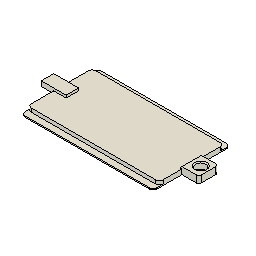
receiver_assembly (Autodesk Fusion 360 archive; units mm, degrees)
design "receiver_battery_door"
Autodesk Fusion 360 part; units mm, degrees
sketch "Sketch1" plane through (0, 0, 0) normal (0, 1, 0) x (1, 0, 0)
  line L0 (26.45, 12.95) -> (-26.45, 12.95)
  line L1 (-26.45, 12.95) -> (-26.45, -12.95)
  line L2 (-26.45, -12.95) -> (26.45, -12.95)
  line L3 (26.45, -12.95) -> (26.45, 12.95)
  line L4 (26.45, 12.95) -> (-26.45, -12.95) construction
  line L5 (-26.45, 12.95) -> (26.45, -12.95) construction
  line L6 (26.45, -15.45) -> (-26.45, -15.45)
  line L7 (-26.45, -15.45) -> (-26.45, 15.45)
  line L8 (-26.45, 15.45) -> (26.45, 15.45)
  line L9 (26.45, 15.45) -> (26.45, -15.45)
  line L10 (26.45, -15.45) -> (-26.45, 15.45) construction
  line L11 (-26.45, -15.45) -> (26.45, 15.45) construction
  dimension "d1" = 52.9
  dimension "d2" = 25.9
  dimension "d9" = 2.5
  constraint horizontal L0
  constraint perpendicular L0 L1
  constraint parallel L0 L2
  constraint parallel L1 L3
  constraint coincident L4 origin
  constraint coincident L5 origin
  constraint horizontal L6
  constraint perpendicular L6 L7
  constraint parallel L6 L8
  constraint parallel L7 L9
  constraint coincident L10 origin
  constraint coincident L11 origin
  constraint coincident L2.end L9
  measures "d1" distance of L0.start L0.end
  measures "d2" distance of L0.end L1.end
  measures "d9" distance of L2 L6
extrude "Extrude1" add sketch "Sketch1" along normal blind 2 contours L0 L1 L2 L3 L7 L9
sketch "Sketch2" plane through (0, 2, 0) normal (0, 1, 0) x (-1, 0, 0)
  line L0 (-26.45, 12.95) -> (-26.45, -12.95)
  line L1 (-26.45, -12.95) -> (26.45, -12.95)
  line L2 (26.45, -12.95) -> (26.45, 12.95)
  line L3 (26.45, 12.95) -> (-26.45, 12.95)
  line L4 (21.45, -2.5) -> (31.45, -2.5)
  line L5 (31.45, -2.5) -> (31.45, 2.5)
  line L6 (31.45, 2.5) -> (21.45, 2.5)
  line L7 (21.45, 2.5) -> (21.45, -2.5)
  line L8 (21.45, -2.5) -> (31.45, 2.5) construction
  line L9 (31.45, -2.5) -> (21.45, 2.5) construction
  point P0 (26.45, 0)
  dimension "d5" = 10
  dimension "d6" = 5
  constraint horizontal L4
  constraint perpendicular L4 L5
  constraint parallel L4 L6
  constraint parallel L5 L7
  constraint coincident L8 P0
  constraint coincident L9 P0
  constraint midpoint L2 P0
  measures "d5" distance of L5.end L6.end
  measures "d6" distance of L4.end L5.end
extrude "Extrude2" add sketch "Sketch2" along normal mid plane 2 contours L2 L4 L5 L6 | L2 L4 L6 L7
extrude "Extrude3" add sketch "Sketch1" along normal blind 0.5
sketch "Sketch3" plane through (0, 0, 0) normal (0, 0, 1) x (1, 0, 0)
  line L0 (26.45, 0.5) -> (-26.45, 0.5)
  line L1 (-26.45, 0.5) -> (-26.45, 2)
  line L2 (-26.45, 2) -> (26.45, 2)
  line L3 (26.45, 2) -> (26.45, 0.5)
  line L4 (26.45, 0) -> (-26.45, 0)
  line L5 (-26.45, 0) -> (-26.45, 0.5)
  line L6 (-26.45, 0.5) -> (26.45, 0.5)
  line L7 (26.45, 0.5) -> (26.45, 0)
  line L8 (26.45, 0) -> (28.55, 0)
  line L9 (28.55, 0) -> (28.55, 2)
  line L10 (28.55, 2) -> (26.45, 2)
  line L11 (26.45, 2) -> (26.45, 0)
  line L12 (28.55, 0) -> (29.55, 0)
  line L13 (29.55, 0) -> (29.55, 5.95)
  line L14 (29.55, 5.95) -> (28.55, 5.95)
  line L15 (28.55, 5.95) -> (28.55, 0)
  line L16 (28.55, 5.95) -> (27.55, 5.95)
  line L17 (27.55, 5.95) -> (27.55, 4.05)
  line L18 (27.55, 4.05) -> (28.55, 4.05)
  line L19 (28.55, 4.05) -> (28.55, 5.95)
  line L20 (28.55, 5.95) -> (27.55, 4.05)
  line L21 (27.55, 5.95) -> (28.55, 4.05) construction
  line L22 (29.55, 5.95) -> (28.4726, 5.3162)
  line L23 (28.4726, 5.3162) -> (31.9726, -0.6338)
  line L24 (31.9726, -0.6338) -> (33.05, 0)
  line L25 (33.05, 0) -> (29.55, 5.95)
  line L26 (33.05, 0) -> (33.05, -1.5)
  line L27 (33.05, -1.5) -> (31.9726, -1.5)
  line L28 (31.9726, -1.5) -> (31.9726, -0.6338)
  line L29 (33.05, 0) -> (29.55, 0) construction
  point P0 (28.05, 5)
  dimension "d12" = 2.1
  dimension "d13" = 2
  dimension "d14" = 1
  dimension "d17" = 3
  dimension "d18" = 1.9
  dimension "d19" = 1
  dimension "d20" = 1.25
  dimension "d21" = 3.5
  dimension "d27" = 1.5
  constraint horizontal L8
  constraint vertical L9
  constraint horizontal L10
  constraint vertical L11
  constraint coincident L4.start L7.end
  constraint horizontal L12
  constraint vertical L13
  constraint horizontal L14
  constraint vertical L15
  constraint horizontal L16
  constraint perpendicular L16 L17
  constraint parallel L16 L18
  constraint parallel L17 L19
  constraint coincident L20 P0
  constraint coincident L21 P0
  constraint coincident L15 L14.end
  constraint coincident L14.end L15.start
  constraint perpendicular L22 L23
  constraint parallel L22 L24
  constraint parallel L23 L25
  constraint vertical L26
  constraint perpendicular L26 L27
  constraint perpendicular L27 L28
  constraint horizontal L29
  measures "d12" distance of L4.start L8.end
  measures "d13" distance of L4.start L2.end
  measures "d14" distance of L8.end L12.end
  measures "d17" distance of L10 P0
  measures "d18" distance of L16.end L17.end
  measures "d19" distance of L17.end L18.end
  measures "d20" distance of L13.end L22.end
  measures "d21" horizontal distance of L12.end L24.end
  measures "d27" distance of L12 L27
sketch "Sketch4" plane through (0, 0, 0) normal (0, 0, 1) x (1, 0, 0)
  line L0 (26.45, 0.5) -> (-26.45, 0.5)
  line L1 (-26.45, 0.5) -> (-26.45, 2)
  line L2 (-26.45, 2) -> (26.45, 2)
  line L3 (26.45, 2) -> (26.45, 0.5)
  line L4 (26.45, 0) -> (-26.45, 0)
  line L5 (-26.45, 0) -> (-26.45, 0.5)
  line L6 (-26.45, 0.5) -> (26.45, 0.5)
  line L7 (26.45, 0.5) -> (26.45, 0)
  line L8 (28.55, 2) -> (26.45, 2)
  line L9 (26.45, 0) -> (28.55, 0)
  line L10 (28.55, 0) -> (29.55, 0)
  line L11 (29.55, 0) -> (29.55, 5.95)
  line L12 (28.55, 0) -> (28.55, 2)
  line L13 (26.45, 0) -> (33.25, 0)
  line L14 (33.25, 0) -> (33.25, 2.8)
  line L15 (33.25, 2.8) -> (26.45, 2.8)
  line L16 (26.45, 2.8) -> (26.45, 0)
  dimension "d30" = 6.8
  dimension "d34" = 2.8
  constraint horizontal L13
  constraint vertical L14
  constraint horizontal L15
  constraint vertical L16
  constraint coincident L4.start L7.end
  measures "d30" distance of L4.start L13.end
  measures "d34" distance of L13.end L14.end
extrude "Extrude6" add sketch "Sketch4" along normal mid plane 7.8 contours L3 L7 L8 L9 L12 L13 L16 | L8 L10 L11 L12 L13 L15 L16 | L11 L13 L14 L15
sketch "Sketch6" plane through (0, 2.8, 0) normal (0, 1, 0) x (-1, 0, 0)
  line L0 (-26.45, -3.9) -> (-26.45, 3.9)
  line L1 (-26.45, 3.9) -> (-33.25, 3.9)
  line L2 (-33.25, 3.9) -> (-33.25, -3.9)
  line L3 (-33.25, -3.9) -> (-26.45, -3.9)
  circle A0 centre (-30, -0.1) radius 2.05
  dimension "d35" = 4.1
  dimension "d38" = 4
  dimension "d39" = 3.55
  measures "d35" diameter of A0
  measures "d38" distance of L1 A0.centre
  measures "d39" distance of L0 A0.centre
extrude "Extrude8" cut sketch "Sketch6" against normal blind 2.5 contours A0
chamfer "Chamfer1" distance 0.4 angle 45 1 edges at (31.9113, 2.8, 0.6413)
chamfer "Chamfer2" distance 0.8 angle 45 1 edges at (26.45, 2, 0)
fillet "Fillet1" radius 1 2 edges at (33.25, 1.4, -3.9) (33.25, 1.4, 3.9)
fillet "Fillet2" radius 1.5 8 edges at (26.45, 1.25, 12.95) (26.45, 0.25, 15.45) (26.45, 1.25, -12.95) (26.45, 0.25, -15.45) (-26.45, 0.25, -15.45) (-26.45, 1.25, -12.95) (-26.45, 0.25, 15.45) (-26.45, 1.25, 12.95)
extrude "Extrude4" [suppressed]
extrude "Extrude5" [suppressed]
